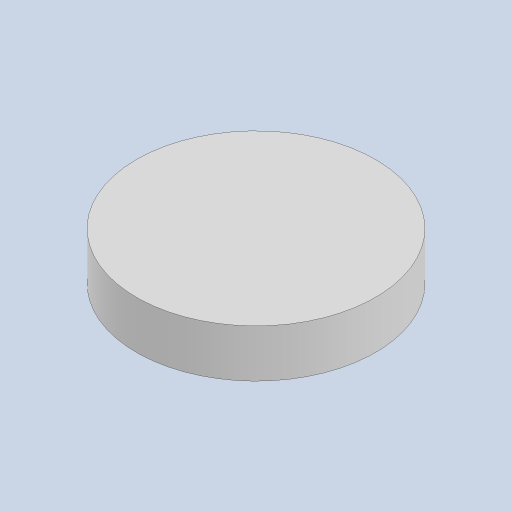
# Autodesk Inventor part: Chalk
Saved by Autodesk Inventor 2024 (Build 280153000, 153)
## iProperties
Created: 2023-11-21
Part Number: Chalk
Material: Generic
Document SubType Name: Modeling
Designer: Greg
Density: 1 g/cm^3
Appearance: Default
Author: Greg
Autodesk Inventor part; units mm, degrees
ref_plane "YZ Plane" through (0, 0, 0) normal (1, 0, 0) x (0, 1, 0)
ref_plane "XZ Plane" through (0, 0, 0) normal (0, 1, 0) x (-1, 0, 0)
ref_plane "XY Plane" through (0, 0, 0) normal (0, 0, 1) x (1, 0, 0)
sketch "Sketch1" plane through (0, 0, 0) normal (0, 1, 0) x (-1, 0, 0)
  circle A0 centre (0, 0) radius 6.35
  dimension "d0" = 12.7
  constraints: 1 centre point, 1 coincident
  measures "d0" diameter of A0
extrude "Extrusion1" add sketch "Sketch1" along normal blind 2.54
sketch "Sketch2" plane through (0, 2.54, 0) normal (0, 1, 0) x (1, 0, 0)
  circle A0 centre (0, 0) radius 11.303
  dimension "d3" = 22.606
  constraints: 1 centre point, 1 coincident
  measures "d3" diameter of A0
extrude "Extrusion2" [suppressed]
sketch "Sketch3" plane through (0, 0, 0) normal (1, 0, 0) x (0, 1, 0)
  line L0 (-73.66, 11.303) -> (-73.66, -11.303) projected
  line L1 (-73.66, 0) -> (-102.235, 0)
  spline S0 degree 4 poles (-102.235, 0) (-102.235, 1.4876) (-95.7427, 4.1779) (-93.4404, 7.0687) (-76.6738, 11.303) (-73.66, 11.303) knots 0 0 0 0 0 0.432698 1 1 1 1 1
  line L2 (-75.2481, 11.303) -> (-72.0719, 11.303) construction
  arc A0 (-72.4281, 11.1502) -> (-74.8919, 11.1502) centre (-73.66, 6.2614) ccw construction
  line L3 (-102.235, -2.1009) -> (-102.235, 2.1009) construction
  arc A1 (-101.7413, 0.8907) -> (-101.7413, -0.8907) centre (-101.1846, 0) ccw construction
  point P0 (0, 0)
  point P1 (-99.695, 2.54)
  point P2 (-92.075, 6.35)
  dimension "d11" = 28.575
  dimension "d12" = 2.54
  dimension "d13" = 2.54
  dimension "d14" = 6.35
  dimension "d15" = 10.16
  constraints: 6 end point, 5 midpoint, 3 horizontal, 2 centre point, 2 point on circle, 2 vertical, 6 other
  measures "d11" distance from line of L1.end L0
  measures "d12" horizontal distance of point (-99.695, 2.54) L1.end
  measures "d13" horizontal distance of point (-99.695, 2.54) L1.end
  measures "d14" vertical distance of L1.end point (-92.075, 6.35)
  measures "d15" horizontal distance of point (-92.075, 6.35) L1.end
revolve "Revolution1" [suppressed]
body "Solid1"
body "Solid2"
